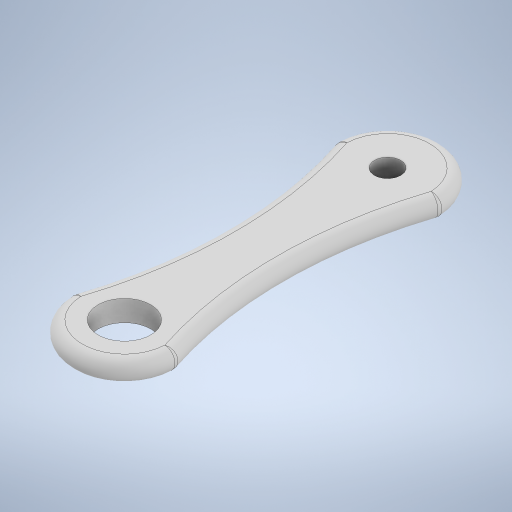
# Autodesk Inventor part: Arm
Saved by Autodesk Inventor 2024 (Build 280153020, 153B)
## iProperties
Created: 2023-09-12
Part Number: Arm
Material: Generic
Document SubType Name: Modeling
Designer: 23also
Density: 1 g/cm^3
Appearance: Default
Author: 23also
Autodesk Inventor part; units mm, degrees
ref_plane "YZ Plane" through (0, 0, 0) normal (1, 0, 0) x (0, 1, 0)
ref_plane "XZ Plane" through (0, 0, 0) normal (0, 1, 0) x (-1, 0, 0)
ref_plane "XY Plane" through (0, 0, 0) normal (0, 0, 1) x (1, 0, 0)
sketch "Sketch1" plane through (0, 0, 0) normal (0, 1, 0) x (-1, 0, 0)
  circle A0 centre (0, 0) radius 10
  circle A1 centre (0, 0) radius 5
  dimension "d0" = 20
  constraints: 2 centre point, 2 coincident
  measures "d0" diameter of A0
extrude "Extrusion1" add sketch "Sketch1" along normal blind 4
sketch "Sketch2" plane through (0, 4, 0) normal (0, 1, 0) x (1, 0, 0)
  circle A0 centre (0, 0) radius 10 projected
  line L0 (-10, 0) -> (10, 0)
  line L1 (10, 0) -> (10, 50)
  line L2 (10, 50) -> (-10, 50)
  line L3 (-10, 50) -> (-10, 0)
  dimension "d3" = 50
  constraints: 8 end point, 2 parallel, 1 horizontal, 1 perpendicular, 2 other
  measures "d3" distance of L1.end L0.end
extrude "Extrusion2" add sketch "Sketch2" against normal blind 4 contours A0 L3 L2 L1
sketch "Sketch3" plane through (0, 4, 0) normal (0, 1, 0) x (1, 0, 0)
  line L0 (-10, 50) -> (10, 50) projected
  circle A0 centre (0, 50) radius 10
  point P0 (0, 0)
  point P1 (-10, 50)
  dimension "d19" = 20
  constraints: 1 midpoint, 3 other
extrude "Extrusion3" add sketch "Sketch3" against normal blind 4 contours A0 L0 picked at (2.78, 54.5572)
sketch "Sketch5" plane through (0, 4, 0) normal (0, 1, 0) x (1, 0, 0)
  arc A0 (-10, 0) -> (10, 0) centre (0, 0) ccw projected
  line L0 (-10, 0) -> (-10, 50) projected
  arc A1 (-10, 0) -> (-10, 50) centre (-86.125, 25) ccw
  line L1 (10, 50) -> (10, 0) projected
  arc A2 (10, 50) -> (10, 0) centre (86.125, 25) ccw
  constraints: 4 point on circle, 2 centre point
extrude "Extrusion4" cut sketch "Sketch5" against normal blind 4
fillet "Fillet1" radius 2 1 edges at (10, 2, -50)
fillet "Fillet2" radius 2 1 edges at (-10, 2, -50)
fillet "Fillet3" radius 2 1 edges at (-10, 2, 0)
fillet "Fillet4" radius 2 1 edges at (10, 2, 0)
sketch "Sketch6" plane through (0, 4, 0) normal (0, 1, 0) x (1, 0, 0)
  arc A0 (9.9929, 50.3757) -> (-9.9929, 50.3757) centre (0, 50) ccw projected
  circle A1 centre (0, 50) radius 2.5
  point P0 (0, 0)
  dimension "d14" = 5
  constraints: 1 centre point, 1 coincident
  measures "d14" diameter of A1
extrude "Extrusion5" cut sketch "Sketch6" against normal blind 4
fillet "Fillet5" radius 2 5 edges at (0, 4, -60) (-9.9754, 4, 0.0258) (0, 4, 10) (9.9754, 4, 0.0258) (6, 4, -25)
fillet "Fillet6" radius 2 5 edges at (0, 0, -60) (6, 0, -25) (9.9754, 0, 0.0258) (0, 0, 10) (-9.9754, 0, 0.0258)
body "Solid1"
